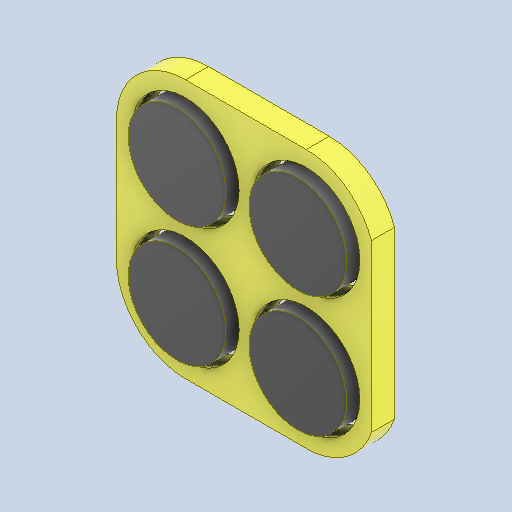
# Autodesk Inventor part: daVinciTool_Aufnahme_ClutchPart
Saved by Autodesk Inventor 2024 (Build 280153000, 153)
## iProperties
Created: 2022-08-12
Part Number: daVinciTool_Aufnahme_ClutchPart
Material: Generisch
Document SubType Name: Modeling
Designer: alexw
Density: 1 g/cm^3
Appearance: Glatt - Gelb
Mass: 32.5123 g
Surface Area: 146.101 cm^2
Volume: 32.5123 cm^3
Author: alexw
Autodesk Inventor part; units mm, degrees
ref_plane "YZ Plane" through (0, 0, 0) normal (1, 0, 0) x (0, 1, 0)
ref_plane "XZ Plane" through (0, 0, 0) normal (0, 1, 0) x (-1, 0, 0)
ref_plane "XY Plane" through (0, 0, 0) normal (0, 0, 1) x (1, 0, 0)
sketch "Skizze1" plane through (0, 0, 0) normal (0, 0, 1) x (1, 0, 0)
  line L0 (-33.75, 33.75) -> (33.75, 33.75)
  line L1 (33.75, 33.75) -> (33.75, -33.75)
  line L2 (33.75, -33.75) -> (-33.75, -33.75)
  line L3 (-33.75, -33.75) -> (-33.75, 33.75)
  circle A0 centre (-15.75, 15.75) radius 18 construction
  circle A1 centre (15.75, 15.75) radius 18 construction
  circle A2 centre (-15.75, -15.75) radius 18 construction
  circle A3 centre (15.75, -15.75) radius 18 construction
  arc A4 (-15.75, 33.75) -> (-33.75, 15.75) centre (-15.75, 15.75) ccw
  arc A5 (33.75, 15.75) -> (15.75, 33.75) centre (15.75, 15.75) ccw
  arc A6 (-33.75, -15.75) -> (-15.75, -33.75) centre (-15.75, -15.75) ccw
  arc A7 (15.75, -33.75) -> (33.75, -15.75) centre (15.75, -15.75) ccw
  circle A8 centre (-15.75, 15.75) radius 14
  circle A9 centre (15.75, 15.75) radius 14
  circle A10 centre (-15.75, -15.75) radius 14
  circle A11 centre (15.75, -15.75) radius 14
  circle A12 centre (-15.75, 15.75) radius 12.75
  circle A13 centre (15.75, 15.75) radius 12.75
  circle A14 centre (-15.75, -15.75) radius 12.75
  circle A15 centre (15.75, -15.75) radius 12.75
  line L4 (33.75, 0) -> (-33.75, 0) construction
  line L5 (0, 33.75) -> (0, -33.75) construction
  line L6 (33.75, 33.75) -> (32.75, 33.75)
  line L7 (32.75, 33.75) -> (32.75, -33.75)
  line L8 (32.75, -33.75) -> (33.75, -33.75)
  line L9 (33.75, -33.75) -> (33.75, 33.75)
  circle A16 centre (0, -30) radius 1 construction
  circle A17 centre (0, 30) radius 1 construction
  line L10 (0, -30) -> (0, 30) construction
  point P0 (0, 0)
  point P1 (0, 0)
  dimension "d0" = 67.5
  dimension "d1" = 67.5
  dimension "d2" = 36
  dimension "d3" = 28
  dimension "d4" = 28
  dimension "d5" = 28
  dimension "d6" = 28
  dimension "d9" = 25.5
  dimension "d14" = 1
  dimension "d17" = 2
  dimension "d18" = 60
  dimension "d19" = 15.75
  constraints: 22 end point, 18 centre point, 16 point on circle, 11 equal radius, 10 coincident, 10 point on line, 8 midpoint, 8 tangent, 4 parallel, 2 horizontal, 2 perpendicular, 1 collinear
  measures "d0" distance between parallel lines of L2 L0
  measures "d1" distance between parallel lines of L3 L1
  measures "d2" diameter of A1
  measures "d3" diameter of A8
  measures "d4" diameter of A9
  measures "d5" diameter of A10
  measures "d6" diameter of A11
  measures "d9" diameter of A12
  measures "d14" distance between parallel lines of L1 L7
  measures "d17" diameter of A16
  measures "d18" distance of L10.start L10.end
  measures "d19" horizontal distance of point (0, 0) A2.centre
extrude "Extrusion1" add sketch "Skizze1" along normal blind 6 contours L0 A5 L7 A7 L2 A6 L3 A4 | A5 L1 A7 L7
extrude "Extrusion2" add sketch "Skizze1" against normal blind 2.5 contours A12 | A13 | A14 | A15
extrude "Extrusion3" add sketch "Skizze1" along normal blind 8.2 contours A12 | A13 | A14 | A15
extrude "Extrusion4" cut sketch "Skizze1" along normal through all contours L0 L1 A5 L7 | A5 L1 A7 L7 | A7 L1 L2 L7
equation "\"d1\" = d0"
equation "\"d3\" = d4"
equation "\"d5\" = d3"
equation "\"d6\" = d4"
